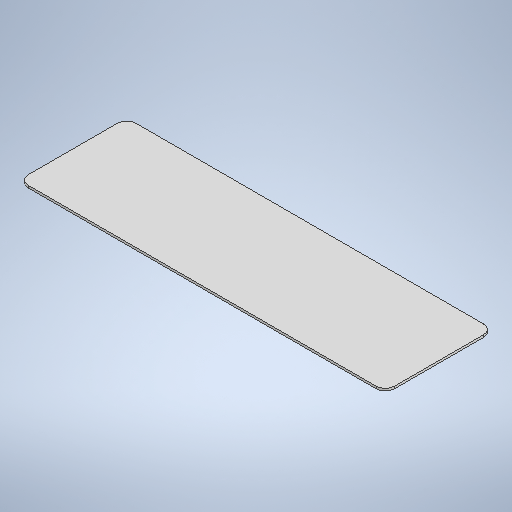
# Autodesk Inventor part: roof
Saved by Autodesk Inventor 2025.2 (Build 292293000, 293)
## iProperties
Created: 2026-06-09
Part Number: roof
Material: Generic
Document SubType Name: Modeling
Designer: AdminOS
Density: 1 g/cm^3
Appearance: Default
Author: AdminOS
Autodesk Inventor part; units mm, degrees
ref_plane "YZ Plane" through (0, 0, 0) normal (1, 0, 0) x (0, 1, 0)
ref_plane "XZ Plane" through (0, 0, 0) normal (0, 1, 0) x (-1, 0, 0)
ref_plane "XY Plane" through (0, 0, 0) normal (0, 0, 1) x (1, 0, 0)
sketch "Sketch1" plane through (0, 0, 0) normal (0, 1, 0) x (-1, 0, 0)
  line L0 (20, 0) -> (780, 0)
  line L1 (800, -20) -> (800, -215)
  line L2 (780, -235) -> (20, -235)
  line L3 (0, -215) -> (0, -20)
  arc A0 (780, -235) -> (800, -215) centre (780, -215) ccw
  arc A1 (800, -20) -> (780, 0) centre (780, -20) ccw
  arc A2 (20, 0) -> (0, -20) centre (20, -20) ccw
  arc A3 (0, -215) -> (20, -235) centre (20, -215) ccw
  point P0 (0, 0)
  point P1 (800, -235)
  point P2 (800, 0)
  point P3 (0, -235)
  dimension "d0" = 800
  dimension "d1" = 235
  dimension "d2" = 20
  constraints: 8 end point, 8 point on circle, 8 point on line, 8 tangent, 4 centre point, 3 equal radius, 2 parallel, 1 horizontal, 1 perpendicular
  measures "d0" distance of point (800, -235) point (0, -235)
  measures "d1" distance of point (800, 0) point (800, -235)
  measures "d2" radius of A0
extrude "Extrusion1" add sketch "Sketch1" along normal blind 5
body "Solid1"
